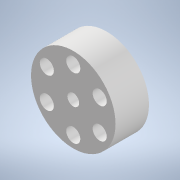
# Autodesk Inventor part: servo flange
Saved by Autodesk Inventor 2021 (Build 250183000, 183)
## iProperties
Created: 2021-11-23
Part Number: servo flange
Material: Generic
Document SubType Name: Modeling
Designer: techv
Density: 1 g/cm^3
Appearance: Default
Author: techv
Autodesk Inventor part; units mm, degrees
ref_plane "YZ Plane" through (0, 0, 0) normal (1, 0, 0) x (0, 1, 0)
ref_plane "XZ Plane" through (0, 0, 0) normal (0, 1, 0) x (-1, 0, 0)
sketch "Sketch1" plane through (0, 0, 0) normal (0, 0, 1) x (1, 0, 0)
  point P0 (0, 0)
sketch "Sketch2" plane through (0, 0, 0) normal (0, 0, 1) x (1, 0, 0)
  circle A0 centre (0, 0) radius 1.25 projected
  circle A1 centre (-5.6292, 3.25) radius 1.5 projected
  circle A2 centre (5.6292, -3.25) radius 1.5 projected
  circle A3 centre (0, 6.5) radius 1.5 projected
  circle A4 centre (-5.6292, -3.25) radius 1.5 projected
  circle A5 centre (0, -6.5) radius 1.5 projected
  circle A6 centre (5.6292, 3.25) radius 1.5 projected
  circle A7 centre (0, 0) radius 9 projected
  point P0 (0, 0)
ref_plane "Work Plane1" through (148.8207, 117.8259, 7.13) normal (0, 0, -1) x (-0.6254, 0.7803, 0)
extrude "Extrusion1" add sketch "Sketch2" along normal up to surface (7.13 mm away)
body "Solid1"
